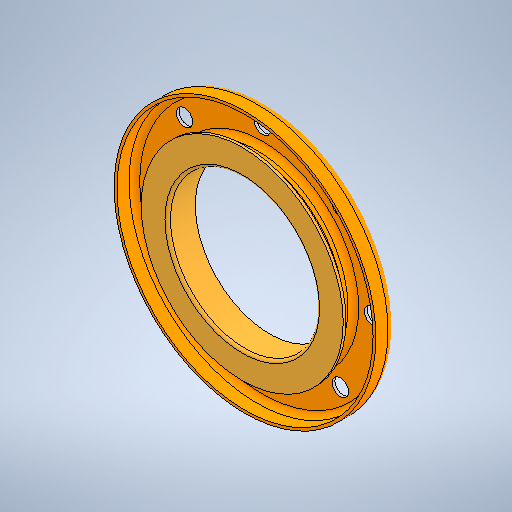
# Autodesk Inventor part: Stamp flange DIN2642-150
Saved by Autodesk Inventor 2025.1 (Build 291241020, 241B)
## iProperties
Created: 2023-02-20
Part Number: Stamp flange DIN2642-150
Material: Stainless Steel
Document SubType Name: Modeling
Designer: user
Density: 8 g/cm^3
Appearance: Semi-Polished
Author: user
Autodesk Inventor part; units mm, degrees
ref_plane "YZ Plane" through (0, 0, 0) normal (1, 0, 0) x (0, 1, 0)
ref_plane "XZ Plane" through (0, 0, 0) normal (0, 1, 0) x (-1, 0, 0)
ref_plane "XY Plane" through (0, 0, 0) normal (0, 0, 1) x (1, 0, 0)
sketch "Sketch1" plane through (0, 0, 0) normal (0, 1, 0) x (-1, 0, 0)
  line L0 (0, 0) -> (0, -45.85397)
  line L1 (-110, 0) -> (-84.15, 0)
  arc A0 (-81.15, -3) -> (-84.15, 0) centre (-84.15, -3) ccw
  line L2 (-81.15, -3) -> (-81.15, -30)
  line L3 (-81.15, -30) -> (-84.15, -30)
  line L4 (-84.15, -30) -> (-84.15, -3)
  arc A1 (-84.15, -3) -> (-84.15, -3) centre (-84.15, -3) ccw
  line L5 (-84.15, -3) -> (-110, -3)
  line L6 (-110, -3) -> (-110, 0)
  point P0 (-97.075, 0)
  dimension "H_cllr" = 30
  dimension "D_ext_tube" = 168.3
  dimension "D_ext_clllr" = 220
  dimension "d26" = 3
  constraints: 14 end point, 6 perpendicular, 4 tangent, 2 centre point, 2 coincident with centre, 2 point on circle, 1 concentric, 1 horizontal, 1 horizontal alignment, 1 midpoint, 1 vertical
  measures "H_cllr" distance from line of L0.start L3
  measures "D_ext_tube" diameter of L4 L0
  measures "D_ext_clllr" diameter of L6 L0
  measures "d26" distance of L2.end L3.end
sketch "Sketch1 outline for Revolution1" plane through (0, 0, 0) normal (0, 1, 0) x (-1, 0, 0)
  arc A0 (-81.15, -3) -> (-84.15, 0) centre (-84.15, -3) ccw
  line L0 (-81.15, -30) -> (-81.15, -3)
  line L1 (-84.15, -30) -> (-81.15, -30)
  line L2 (-84.15, -3) -> (-84.15, -30)
  line L3 (-110, -3) -> (-84.15, -3)
  line L4 (-110, 0) -> (-110, -3)
  line L5 (-84.15, 0) -> (-110, 0)
revolve "Revolution1" add sketch "Sketch1 outline for Revolution1" angle 360 about axis through (0, 0, 0) along (0, 0, -1)
sketch "Sketch2" plane through (0, 0, 0) normal (0, 1, 0) x (-1, 0, 0)
  line L0 (0, 0) -> (0, -50.951284)
  line L1 (-86.5, -6) -> (-90.1875, -6)
  arc A0 (-90.1875, -6) -> (-96, -11.8125) centre (-90.1875, -11.8125) ccw
  line L2 (-96, -11.8125) -> (-96, -16.1875)
  arc A1 (-104.8125, -25) -> (-96, -16.1875) centre (-104.8125, -16.1875) ccw
  line L3 (-104.8125, -25) -> (-133.6875, -25)
  arc A2 (-142.5, -16.1875) -> (-133.6875, -25) centre (-133.6875, -16.1875) ccw
  line L4 (-142.5, -16.1875) -> (-142.5, -3)
  line L5 (-142.5, -3) -> (-139.5, -3)
  line L6 (-139.5, -3) -> (-139.5, -16.1875)
  arc A3 (-139.5, -16.1875) -> (-133.6875, -22) centre (-133.6875, -16.1875) ccw
  line L7 (-133.6875, -22) -> (-104.8125, -22)
  arc A4 (-104.8125, -22) -> (-99, -16.1875) centre (-104.8125, -16.1875) ccw
  line L8 (-99, -16.1875) -> (-99, -11.8125)
  arc A5 (-90.1875, -3) -> (-99, -11.8125) centre (-90.1875, -11.8125) ccw
  line L9 (-90.1875, -3) -> (-86.5, -3)
  line L10 (-86.5, -3) -> (-86.5, -6)
  point P0 (-141, -3)
  point P1 (-88.34375, -3)
  dimension "d8" = 3
  dimension "Thknss_lpd" = 3
  dimension "d10" = 5.8125
  dimension "H_lpd" = 22
  dimension "D_ext_lpd" = 285
  dimension "d_inn_lpd" = 173
  dimension "d2_inn_lpd" = 192
  dimension "d23" = 46.5
  constraints: 22 end point, 12 point on circle, 12 tangent, 8 perpendicular, 6 centre point, 3 concentric, 2 equal radius, 2 midpoint, 2 point on line, 1 horizontal, 1 horizontal alignment, 1 vertical
  measures "d8" distance from line of L0.start L9
  measures "Thknss_lpd" distance of L9.end L1.start
  measures "d10" radius of A0
  measures "H_lpd" distance between parallel lines of L5 L3
  measures "D_ext_lpd" diameter of L4 L0
  measures "d_inn_lpd" diameter of L10 L0
  measures "d2_inn_lpd" diameter of L2 L0
  measures "d23" distance between parallel lines of L4 L2
revolve "Revolution2" add sketch "Sketch2" angle 360 about axis through (0, 0, 0) along (0, 0, -1)
sketch "Sketch3" plane through (0, 0, 0) normal (0, 0, 1) x (1, 0, 0)
  circle A0 centre (120, 0) radius 9
  line L0 (0, 0) -> (0, 123.830608)
  dimension "hl_d" = 18
  dimension "D_hl_c" = 240
  constraints: 2 end point, 1 centre point, 1 horizontal alignment, 1 vertical
  measures "hl_d" diameter of A0
  measures "D_hl_c" diameter of A0.centre L0
extrude "Extrusion1" cut sketch "Sketch3" against normal through all
pattern_circular "Circular Pattern1" count 8 over 360 about axis through (0, 0, -10) along (0, 0, 1) of "Extrusion1"
equation "\"d26\" = Thknss_lpd"
equation "\"d8\" = Thknss_cllr"
equation "\"d10\" = 0.125 * d23"
equation "\"Thknss_cllr\" = 3"
body "Solid1"
